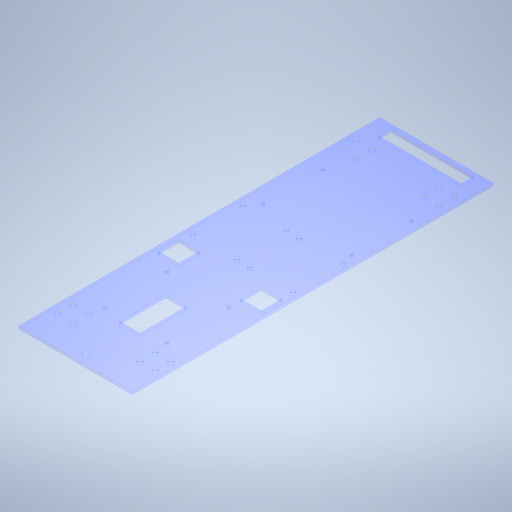
# Autodesk Inventor part: plat
Saved by Autodesk Inventor 2023 (Build 270158000, 158)
## iProperties
Created: 2023-04-12
Part Number: plat
Material: Nylon 6/6
Document SubType Name: Modeling
Designer: LAB-505
Density: 1.13 g/cm^3
Appearance: Clear - Blue
Mass: 119.82 g
Surface Area: 762.009 cm^2
Volume: 106.035 cm^3
Author: LAB-505
Autodesk Inventor part; units mm, degrees
ref_plane "YZ Plane" through (0, 0, 0) normal (1, 0, 0) x (0, 1, 0)
ref_plane "XZ Plane" through (0, 0, 0) normal (0, 1, 0) x (-1, 0, 0)
ref_plane "XY Plane" through (0, 0, 0) normal (0, 0, 1) x (1, 0, 0)
sketch "Sketch1" plane through (0, 0, 0) normal (0, 1, 0) x (-1, 0, 0)
  line L0 (55, 175) -> (-55, 175)
  line L1 (-55, 175) -> (-55, -175)
  line L2 (-55, -175) -> (55, -175)
  line L3 (55, -175) -> (55, 175)
  line L4 (55, 175) -> (-55, -175) construction
  line L5 (-55, 175) -> (55, -175) construction
  point P0 (0, 0)
  dimension "d0" = 110
  dimension "d1" = 350
  constraints: 12 end point, 2 midpoint, 2 parallel, 1 horizontal, 1 perpendicular
  measures "d0" distance of L2.end L1.end
  measures "d1" distance of L1.end L0.end
extrude "Extrusion1" add sketch "Sketch1" along normal blind 3
sketch "Sketch2" plane through (0, 3, 0) normal (0, 1, 0) x (1, 0, 0)
  circle A0 centre (-47.5, 145) radius 2.5
  circle A1 centre (-32.5, 145) radius 2.5
  circle A2 centre (-47.5, 130) radius 2.5
  circle A3 centre (-32.5, 130) radius 2.5
  circle A4 centre (47.5, 145) radius 2.5
  circle A5 centre (32.5, 145) radius 2.5
  circle A6 centre (32.5, 130) radius 2.5
  circle A7 centre (47.5, 130) radius 2.5
  circle A8 centre (-47.5, -145) radius 2.5
  circle A9 centre (-32.5, -145) radius 2.5
  circle A10 centre (-47.5, -130) radius 2.5
  circle A11 centre (-32.5, -130) radius 2.5
  circle A12 centre (47.5, -130) radius 2.5
  circle A13 centre (32.5, -130) radius 2.5
  circle A14 centre (32.5, -145) radius 2.5
  circle A15 centre (47.5, -145) radius 2.5
  point P0 (0, 0)
  dimension "d4" = 5
  dimension "d5" = 5
  dimension "d6" = 5
  dimension "d7" = 5
  dimension "d8" = 5
  dimension "d9" = 5
  dimension "d10" = 5
  dimension "d11" = 5
  dimension "d12" = 5
  dimension "d13" = 5
  dimension "d14" = 5
  dimension "d15" = 5
  dimension "d16" = 5
  dimension "d17" = 5
  constraints: 16 centre point
  measures "d4" diameter of A0
  measures "d5" diameter of A1
  measures "d6" diameter of A2
  measures "d7" diameter of A3
  measures "d8" diameter of A4
  measures "d9" diameter of A5
  measures "d10" diameter of A6
  measures "d11" diameter of A7
  measures "d12" diameter of A8
  measures "d13" diameter of A9
  measures "d14" diameter of A10
  measures "d15" diameter of A12
  measures "d16" diameter of A13
  measures "d17" diameter of A14
extrude "Extrusion2" cut sketch "Sketch2" against normal blind 77.9625
sketch "Sketch3" plane through (0, 3, 0) normal (0, 1, 0) x (1, 0, 0)
  circle A0 centre (0, -165) radius 3
  point P0 (0, 0)
  dimension "d20" = 6
  constraints: 1 centre point
  measures "d20" diameter of A0
extrude "Extrusion3" cut sketch "Sketch3" against normal blind 75.725
sketch "Sketch4" plane through (0, 3, 0) normal (0, 1, 0) x (1, 0, 0)
  circle A0 centre (-40.0264, 38.7331) radius 1.375
  circle A1 centre (45.9736, 38.7331) radius 1.375
  circle A2 centre (45.9736, -19.2669) radius 1.375
  circle A3 centre (-40.0264, -19.2669) radius 1.375
  line L0 (-50.0264, -35.6669) -> (-50.0264, 42.1331)
  line L1 (-49.4264, 42.7331) -> (49.3736, 42.7331)
  line L2 (49.9736, 42.1331) -> (49.9736, -35.6669)
  line L3 (39.4736, -37.5169) -> (48.4736, -37.5169)
  line L4 (49.3736, -36.2669) -> (-49.4264, -36.2669)
  circle A4 centre (-40.0264, 46.7331) radius 1.375
  circle A5 centre (45.9736, 46.7331) radius 1.375
  circle A6 centre (45.9736, 104.7331) radius 1.375
  circle A7 centre (-40.0264, 104.7331) radius 1.375
  line L5 (-50.0264, 121.1331) -> (-50.0264, 43.3331)
  line L6 (49.9736, 43.3331) -> (49.9736, 121.1331)
  line L7 (39.4736, 122.9831) -> (48.4736, 122.9831)
  line L8 (49.3736, 121.7331) -> (-49.4264, 121.7331)
  point P0 (0, 0)
  point P1 (0, 85.4662)
  constraints: 18 end point, 13 symmetric about line, 8 centre point, 4 other
extrude "Extrusion4" cut sketch "Sketch4" against normal blind 476.725 contours A4 | A5 | A6 | A7
sketch "Sketch7" plane through (0, 0, 0) normal (0, -1, 0) x (1, 0, 0)
  circle A0 centre (30.058, 56.5394) radius 1.5
  circle A1 centre (30.058, 116.5394) radius 1.5
  circle A2 centre (-29.942, 56.5394) radius 1.5
  circle A3 centre (-29.942, 116.5394) radius 1.5
  circle A4 centre (21.6655, 65.4546) radius 1.319
  circle A5 centre (21.6655, 108.4546) radius 1.319
  circle A6 centre (-21.3345, 65.4546) radius 1.319
  circle A7 centre (-21.3345, 108.4546) radius 1.319
  line L0 (35.058, 51.5394) -> (35.058, 121.5394)
  line L1 (35.058, 121.5394) -> (-34.942, 121.5394)
  line L2 (-34.942, 121.5394) -> (-34.942, 51.5394)
  line L3 (-34.942, 51.5394) -> (35.058, 51.5394)
  point P0 (0, 0)
  constraints: 8 centre point, 8 end point
extrude "Extrusion6" cut sketch "Sketch7" against normal blind 157.6375 contours A0 | A1 | A2 | A3
sketch "Sketch8" plane through (0, 0, 0) normal (0, -1, 0) x (1, 0, 0)
  circle A0 centre (-6.448, -35.5938) radius 2
  circle A1 centre (-6.4424, -28.5958) radius 2
  circle A2 centre (-48.518, -35.5603) radius 2
  circle A3 centre (-48.5124, -28.5623) radius 2
  circle A4 centre (-48.5025, -16.1623) radius 2
  circle A5 centre (-48.4797, 12.4797) radius 2
  circle A6 centre (-6.4097, 12.4462) radius 2
  line L0 (-51.4396, 18.8876) -> (-3.4396, 18.8494)
  line L1 (-51.485, -38.1124) -> (-51.4396, 18.8876)
  line L2 (-3.4396, 18.8494) -> (-3.485, -38.1506)
  line L3 (-3.485, -38.1506) -> (-51.485, -38.1124)
  circle A7 centre (48.5726, -35.5524) radius 2
  circle A8 centre (48.5782, -28.5544) radius 2
  circle A9 centre (6.5026, -35.5189) radius 2
  circle A10 centre (6.5082, -28.5209) radius 2
  circle A11 centre (6.5181, -16.1209) radius 2
  circle A12 centre (6.5409, 12.5211) radius 2
  circle A13 centre (48.6109, 12.4876) radius 2
  line L4 (3.581, 18.929) -> (51.581, 18.8908)
  line L5 (3.5356, -38.071) -> (3.581, 18.929)
  line L6 (51.581, 18.8908) -> (51.5356, -38.1092)
  line L7 (51.5356, -38.1092) -> (3.5356, -38.071)
  point P0 (0, 0)
  point P1 (0.4743, -5.9122)
  constraints: 16 end point, 14 centre point
extrude "Extrusion7" cut sketch "Sketch8" against normal blind 73.5 contours A0 | A2 | A5 | A6 | A7 | A9 | A12 | A13
sketch "Sketch9" plane through (0, 3, 0) normal (0, 1, 0) x (1, 0, 0)
  line L0 (30, -45) -> (50, -45)
  line L1 (50, -45) -> (50, -25)
  line L2 (50, -25) -> (30, -25)
  line L3 (30, -25) -> (30, -45)
  line L4 (30, -45) -> (50, -25) construction
  line L5 (50, -45) -> (30, -25) construction
  line L6 (-50, -45) -> (-30, -45)
  line L7 (-30, -45) -> (-30, -25)
  line L8 (-30, -25) -> (-50, -25)
  line L9 (-50, -25) -> (-50, -45)
  line L10 (-50, -45) -> (-30, -25) construction
  line L11 (-30, -45) -> (-50, -25) construction
  point P0 (0, 0)
  point P1 (40, -35)
  point P2 (-40, -35)
  dimension "d31" = 20
  dimension "d32" = 20
  dimension "d33" = 20
  constraints: 24 end point, 4 midpoint, 4 parallel, 2 horizontal, 2 perpendicular
  measures "d31" distance of L2.end L1.end
  measures "d32" distance of L1.end L0.end
  measures "d33" distance of L8.end L7.end
extrude "Extrusion8" cut sketch "Sketch9" against normal blind 163.0375
sketch "Sketch10" plane through (0, 3, 0) normal (0, 1, 0) x (1, 0, 0)
  line L0 (40, 159) -> (-40, 159)
  line L1 (-40, 159) -> (-40, 171)
  line L2 (-40, 171) -> (40, 171)
  line L3 (40, 171) -> (40, 159)
  line L4 (40, 159) -> (-40, 171) construction
  line L5 (-40, 159) -> (40, 171) construction
  point P0 (0, 0)
  point P1 (0, 165)
  dimension "d36" = 80
  dimension "d37" = 12
  constraints: 12 end point, 2 midpoint, 2 parallel, 1 horizontal, 1 perpendicular
  measures "d36" distance of L1.end L2.end
  measures "d37" distance of L0.end L1.end
extrude "Extrusion9" cut sketch "Sketch10" against normal blind 159.225
sketch "Sketch11" plane through (0, 3, 0) normal (0, 1, 0) x (1, 0, 0)
  line L0 (10, -122.5215) -> (-10, -122.5215)
  line L1 (-10, -122.5215) -> (-10, -77.5215)
  line L2 (-10, -77.5215) -> (10, -77.5215)
  line L3 (10, -77.5215) -> (10, -122.5215)
  line L4 (10, -122.5215) -> (-10, -77.5215) construction
  line L5 (-10, -122.5215) -> (10, -77.5215) construction
  point P0 (0, 0)
  point P1 (0, -100.0215)
  dimension "d40" = 20
  dimension "d41" = 45
  constraints: 12 end point, 2 midpoint, 2 parallel, 1 horizontal, 1 perpendicular
  measures "d40" distance of L1.end L2.end
  measures "d41" distance of L0.end L1.end
extrude "Extrusion10" cut sketch "Sketch11" against normal blind 113.825
body "Solid1"
